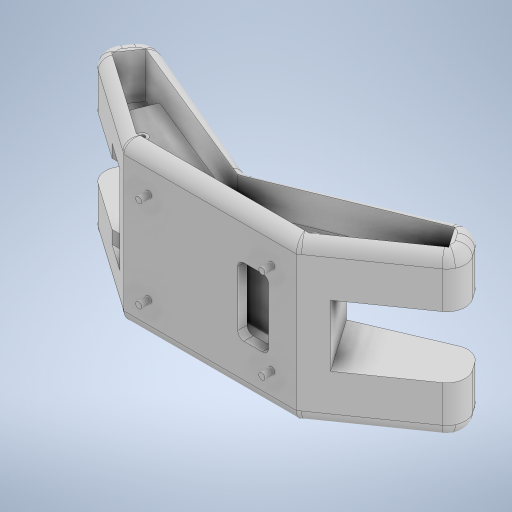
# Autodesk Inventor part: podvozek
Saved by Autodesk Inventor 2024 (Build 280153000, 153)
## iProperties
Created: 2024-03-05
Part Number: podvozek
Material: Všeobecné
Document SubType Name: Modeling
Designer: Game
Density: 1 g/cm^3
Appearance: Výchozí
Author: Game
Autodesk Inventor part; units mm, degrees
ref_plane "XZ Plane" through (0, 0, 0) normal (0, 1, 0) x (-1, 0, 0)
ref_plane "XY Plane" through (0, 0, 0) normal (0, 0, 1) x (1, 0, 0)
sketch "Náčrt1" plane through (0, 0, 0) normal (0, 0, 1) x (1, 0, 0)
  line L0 (-70, 45) -> (70, 45)
  line L1 (70, 45) -> (70, -45)
  line L2 (70, -45) -> (-70, -45)
  line L3 (-70, -45) -> (-70, 45)
  line L4 (-70, 45) -> (70, -45) construction
  line L5 (70, 45) -> (-70, -45) construction
  point P0 (0, 0)
  dimension "d0" = 140
  dimension "d1" = 90
  constraints: 12 end point, 2 midpoint, 2 parallel, 1 horizontal, 1 perpendicular
  measures "d0" distance of L1.end L2.end
  measures "d1" distance of L0.end L1.end
extrude "Vysunutí1" add sketch "Náčrt1" along normal blind 30
sketch "Náčrt2" plane through (-70, -45, 0) normal (-1, 0, 0) x (0, 0, 1)
  line L0 (7.5, 80.5) -> (22.5, 80.5)
  line L1 (22.5, 80.5) -> (22.5, 9.5)
  line L2 (22.5, 9.5) -> (7.5, 9.5)
  line L3 (7.5, 9.5) -> (7.5, 80.5)
  line L4 (7.5, 80.5) -> (22.5, 9.5) construction
  line L5 (22.5, 80.5) -> (7.5, 9.5) construction
  point P0 (0, 45)
  point P1 (15, 45)
  dimension "d4" = 15
  dimension "d5" = 71
  constraints: 12 end point, 2 midpoint, 2 parallel, 1 horizontal, 1 perpendicular
  measures "d4" distance of L1.end L2.end
  measures "d5" distance of L0.end L1.end
extrude "Vysunutí2" cut sketch "Náčrt2" against normal blind 132
sketch "Náčrt3" plane through (0, 0, 30) normal (0, 0, 1) x (1, 0, 0)
  line L0 (50, 37) -> (-50, 37)
  line L1 (-50, 37) -> (-50, -37)
  line L2 (-50, -37) -> (50, -37)
  line L3 (50, -37) -> (50, 37)
  line L4 (50, 37) -> (-50, -37) construction
  line L5 (-50, 37) -> (50, -37) construction
  circle A0 centre (50, -37) radius 2.5
  circle A1 centre (50, 37) radius 2.5
  circle A2 centre (-50, -37) radius 2.5
  circle A3 centre (-50, 37) radius 2.5
  point P0 (0, 0)
  dimension "d8" = 100
  dimension "d9" = 74
  dimension "d10" = 5
  dimension "d13" = 74
  dimension "d16" = 100
  constraints: 12 end point, 4 centre point, 2 horizontal, 2 midpoint, 2 parallel, 1 coincident, 1 perpendicular, 1 vertical, 6 other
  measures "d8" distance of L2.end L1.end
  measures "d9" distance of L1.end L0.end
  measures "d10" diameter of A0
  measures "d13" distance of A0.centre A1.centre
  measures "d16" distance of A0.centre A2.centre
extrude "Vysunutí3" add sketch "Náčrt3" along normal blind 8 contours A3 L1 L0 | L0 L1 A3 | A1 L3 L0 | L0 L3 A1 | A2 L2 L1 | L1 L2 A2 | A0 L2 L3 | L3 L2 A0
sketch "Náčrt7" plane through (-70, 45, 0) normal (0, 1, 0) x (1, 0, 0)
  line L0 (140, 0) -> (140, -30) projected
  line L1 (140, -30) -> (221.9152, 27.3576)
  line L2 (140, -30) -> (240, -30) construction
  line L3 (221.9152, 27.3576) -> (201.84, 56.028)
  line L4 (201.84, 56.028) -> (70, 0)
  line L5 (0, -30) -> (140, -30) projected
  line L6 (0, -30) -> (-81.9152, 27.3576)
  line L7 (0, -30) -> (100, -30) construction
  line L8 (-81.9152, 27.3576) -> (-61.84, 56.028)
  line L9 (-61.84, 56.028) -> (70, 0)
  dimension "d39" = 100
  dimension "d40" = 35
  dimension "d41" = 35
  dimension "d42" = 100
  dimension "d43" = 145
  dimension "d44" = 35
  constraints: 16 end point, 2 equal length, 2 horizontal, 2 perpendicular
  measures "d39" distance of L0.end L1.end
  measures "d40" angle of L2 L1
  measures "d41" distance of L1.end L3.end
  measures "d42" distance of L5.start L6.end
  measures "d43" angle of L7 L6
  measures "d44" distance of L6.end L8.end
extrude "Vysunutí7" add sketch "Náčrt7" along normal blind 20 and the other way blind 110
sketch "Náčrt8" plane through (-70, -65, 30) normal (-0.5735764, 0, 0.819152) x (0.819152, 0, 0.5735764)
  line L0 (-180, 90) -> (-20, 90)
  line L1 (-20, 90) -> (-20, 40)
  line L2 (-20, 40) -> (-180, 40)
  line L3 (-180, 40) -> (-180, 90)
  line L4 (-100, 0) -> (-100, 130) projected
  line L5 (-180, 90) -> (-20, 40) construction
  line L6 (-20, 90) -> (-180, 40) construction
  point P0 (40.1334, 65)
  point P1 (-100, 65)
  point P2 (-100, 40)
  point P3 (-100, 90)
  dimension "d49" = 160
  dimension "d50" = 50
  constraints: 12 end point, 3 midpoint, 2 parallel, 1 horizontal, 1 perpendicular
  measures "d49" distance of L1.end L2.end
  measures "d50" distance of L0.end L1.end
extrude "Vysunutí8" cut sketch "Náčrt8" against normal blind 100
sketch "Náčrt9" plane through (151.9152, -65, -27.3576) normal (0.5735764, 0, 0.819152) x (0.819152, 0, -0.5735764)
  line L0 (-80, 40) -> (80, 40)
  line L1 (80, 40) -> (80, 90)
  line L2 (80, 90) -> (-80, 90)
  line L3 (-80, 90) -> (-80, 40)
  line L4 (0, 130) -> (0, 0) projected
  line L5 (-80, 40) -> (80, 90) construction
  line L6 (80, 40) -> (-80, 90) construction
  point P0 (-140.1334, 65)
  point P1 (0, 65)
  point P2 (0, 40)
  point P3 (0, 90)
  dimension "d53" = 160
  dimension "d54" = 50
  constraints: 12 end point, 3 midpoint, 2 parallel, 1 horizontal, 1 perpendicular
  measures "d53" distance of L2.end L1.end
  measures "d54" distance of L1.end L0.end
extrude "Vysunutí9" cut sketch "Náčrt9" against normal blind 100
ref_plane "Pracovní rovina1" through (-120, 0, 0) normal (1, 0, 0) x (0, 1, 0)
sketch "Náčrt11" plane through (-120, 0, 0) normal (1, 0, 0) x (0, 1, 0)
  line L0 (35.5, 22.5) -> (-35.5, 22.5)
  line L1 (-35.5, 22.5) -> (-35.5, 7.5)
  line L2 (-35.5, 7.5) -> (35.5, 7.5)
  line L3 (35.5, 7.5) -> (35.5, 22.5)
  line L4 (35.5, 22.5) -> (-35.5, 7.5) construction
  line L5 (-35.5, 22.5) -> (35.5, 7.5) construction
  point P0 (0, 0)
  point P1 (0, 15)
  dimension "d58" = 71
  dimension "d59" = 15
  constraints: 12 end point, 2 midpoint, 2 parallel, 1 horizontal, 1 perpendicular
  measures "d58" distance of L2.end L1.end
  measures "d59" distance of L1.end L0.end
extrude "Vysunutí10" cut sketch "Náčrt11" along normal blind 170
sketch "Náčrt12" plane through (-70, -65, 0) normal (0, -1, 0) x (1, 0, 0)
  line L0 (0, 20) -> (-66.8295, -26.7945)
  line L1 (0, 20) -> (81.5838, 20) construction
  line L2 (-66.8295, -26.7945) -> (-55.358, -43.1776)
  line L3 (-55.358, -43.1776) -> (70.0734, 7.5)
  line L4 (-32.1333, 7.5) -> (120, 7.5) projected
  line L5 (-55.358, -43.1776) -> (79.9241, -43.1776) construction
  line L6 (70.0734, 7.5) -> (195.5047, -43.1775)
  line L7 (70.0734, 7.5) -> (205.3554, 7.5) construction
  line L8 (0, 20) -> (140, 20)
  line L9 (140, 20) -> (206.9279, -26.8634)
  line L10 (206.9279, -26.8634) -> (195.5047, -43.1775)
  point P0 (70, 0)
  dimension "d62" = 145
  dimension "d63" = 20
  dimension "d64" = 22
  dimension "d65" = 135.282
  dimension "d66" = 22
  dimension "d67" = 145
  constraints: 20 end point, 4 horizontal, 3 equal length, 2 perpendicular, 1 point on line
  measures "d62" angle of L0 L1
  measures "d63" distance of L0.end L2.end
  measures "d64" angle of L5 L3
  measures "d65" distance of L3.end L6.end
  measures "d66" angle of L6 L7
  measures "d67" angle of L8 L9
extrude "Vysunutí11" cut sketch "Náčrt12" against normal blind 25
sketch "Náčrt13" plane through (-70, 65, 0) normal (0, 1, 0) x (1, 0, 0)
  line L0 (-66.8295, 26.7945) -> (0, -20) projected
  line L1 (0, -20) -> (-66.8295, 26.7945)
  line L2 (70.0734, -7.5) -> (-55.358, 43.1776) projected
  line L3 (-66.8295, 26.7945) -> (-55.358, 43.1776)
  line L4 (-55.358, 43.1776) -> (70, -7.6373)
  line L5 (70, -7.6373) -> (195.5048, 43.1776)
  line L6 (195.5047, 43.1775) -> (70.0734, -7.5) projected
  line L7 (206.9279, 26.8634) -> (195.5047, 43.1775) projected
  line L8 (0, -20) -> (140, -20) projected
  line L9 (206.9279, 26.8634) -> (140, -20)
  line L10 (140, -20) -> (0, -20)
  point P0 (70, 0)
  constraints: 12 end point, 2 collinear, 1 perpendicular, 1 point on line
extrude "Vysunutí12" cut sketch "Náčrt13" against normal blind 25 contours L3 L4 L5 L7 L9 L8 L0
sketch "Náčrt14" plane through (0, 0, 30) normal (0, 0, 1) x (1, 0, 0)
  line L0 (47.5, 27.5) -> (22.5, 27.5)
  line L1 (22.5, 27.5) -> (22.5, -27.5)
  line L2 (22.5, -27.5) -> (47.5, -27.5)
  line L3 (47.5, -27.5) -> (47.5, 27.5)
  line L4 (47.5, 27.5) -> (22.5, -27.5) construction
  line L5 (22.5, 27.5) -> (47.5, -27.5) construction
  point P0 (0, 0)
  point P1 (35, 0)
  dimension "d72" = 25
  dimension "d73" = 55
  constraints: 12 end point, 2 midpoint, 2 parallel, 1 horizontal, 1 perpendicular
  measures "d72" distance of L2.end L1.end
  measures "d73" distance of L1.end L0.end
extrude "Vysunutí13" cut sketch "Náčrt14" against normal blind 20
fillet "Zaoblení1" radius 5 4 edges at (47.5, 27.5, 26.25) (47.5, -27.5, 26.25) (22.5, 27.5, 26.25) (22.5, -27.5, 26.25)
fillet "Zaoblení2" radius 10 1 edges at (0, 0, 0)
sketch "Náčrt17" plane through (-70, -40, 0) normal (0, -1, 0) x (1, 0, 0)
  line L0 (-55.358, -43.1776) -> (-66.8295, -26.7945) projected
  line L1 (70.0734, 7.5) -> (-55.358, -43.1776) projected
  line L2 (-66.8295, -26.7945) -> (-55.358, -43.1776)
  line L3 (-55.358, -43.1776) -> (-36.8143, -35.6854)
  line L4 (-36.8143, -35.6854) -> (-46.2332, -12.3728)
  line L5 (-66.8295, -26.7945) -> (0, 20) projected
  line L6 (-46.2332, -12.3728) -> (-66.8295, -26.7945)
  line L7 (195.5047, -43.1775) -> (70.0734, 7.5) projected
  line L8 (195.5047, -43.1775) -> (176.961, -35.6854)
  line L9 (206.9279, -26.8634) -> (195.5047, -43.1775) projected
  line L10 (195.5047, -43.1775) -> (206.9279, -26.8634)
  line L11 (206.9279, -26.8634) -> (140, 20) projected
  line L12 (176.961, -35.6854) -> (187.1443, -10.4809)
  line L13 (176.961, -35.6854) -> (204.1449, -35.6854) construction
  line L14 (206.9279, -26.8634) -> (186.3476, -12.4529)
  point P0 (70, 0)
  dimension "d78" = 20
  dimension "d79" = 90
  dimension "d82" = 20
  dimension "d83" = 68
  constraints: 18 end point, 5 point on line, 1 collinear, 1 equal length, 1 horizontal, 1 perpendicular
  measures "d78" distance of L0.start L3.end
  measures "d79" angle of L4 L3
  measures "d82" distance of L7.start L8.end
  measures "d83" angle of L13 L12
extrude "Vysunutí14" cut sketch "Náčrt17" against normal blind 12
sketch "Náčrt18" plane through (-70, 40, 0) normal (0, 1, 0) x (1, 0, 0)
  line L0 (70, -7.6373) -> (195.5047, 43.1775) projected
  line L1 (195.5047, 43.1775) -> (176.9665, 35.6717)
  line L2 (176.9665, 35.6717) -> (186.3631, 12.4638)
  line L3 (206.9279, 26.8634) -> (140, -20) projected
  line L4 (186.3631, 12.4638) -> (206.9279, 26.8634)
  line L5 (206.9279, 26.8634) -> (195.5047, 43.1775)
  line L6 (-55.358, 43.1776) -> (70, -7.6373) projected
  line L7 (-55.358, 43.1776) -> (-36.8229, 35.6642)
  line L8 (-55.358, 43.1776) -> (70, -7.6373) projected
  line L9 (-36.8229, 35.6642) -> (-46.2574, 12.3898)
  line L10 (0, -20) -> (-66.8295, 26.7945) projected
  line L11 (-46.2574, 12.3898) -> (-66.8295, 26.7945)
  line L12 (-66.8295, 26.7945) -> (-55.358, 43.1776)
  point P0 (70, 0)
  dimension "d84" = 20
  dimension "d85" = 90
  dimension "d86" = 20
  dimension "d87" = 90
  constraints: 16 end point, 4 point on line, 2 collinear, 2 perpendicular
  measures "d84" distance of L0.end L1.end
  measures "d85" angle of L2 L1
  measures "d86" distance of L6.start L7.end
  measures "d87" angle of L7 L9
extrude "Vysunutí15" cut sketch "Náčrt18" against normal blind 12
sketch "Náčrt19" plane through (-70, -40, 0) normal (0, -1, 0) x (1, 0, 0)
  circle A0 centre (105, 15) radius 4
  point P0 (70, 0)
  dimension "d90" = 8
  constraints: 1 centre point
  measures "d90" diameter of A0
extrude "Vysunutí16" cut sketch "Náčrt19" against normal blind 100
fillet "Zaoblení3" radius 15 8 edges at (-151.9152, -45, -27.3576) (-131.84, -45, -56.028) (-151.9152, 45, -27.3576) (-131.84, 45, -56.028) (131.84, 45, -56.028) (131.84, -45, -56.028) (151.9152, -45, -27.3576) (151.9152, 45, -27.3576)
fillet "Zaoblení4" radius 10 24 edges at (0, 65, 30) (-145.7964, 65, -28.4366) (-141.0608, 65, -42.8593) (-130.6544, 65, -51.8898) (-62.2836, 65, -26.4686) (0, 65, -0.8655) (62.2836, 65, -26.4686) (130.6544, 65, -51.8898) (141.0608, 65, -42.8593) (145.7964, 65, -28.4366) (104.814, 65, 5.623) (-104.814, 65, 5.623) (-145.7964, -65, -28.4366) (-141.0608, -65, -42.8593) (-130.6544, -65, -51.8898) (-62.2836, -65, -26.4686) (0, -65, -0.8655) (62.2836, -65, -26.4686) (130.6544, -65, -51.8898) (141.0608, -65, -42.8593) (145.7964, -65, -28.4366) (104.814, -65, 5.623) (-104.814, -65, 5.623) (0, -65, 30)
sketch "Náčrt20" plane through (-70, -40, 0) normal (0, -1, 0) x (1, 0, 0)
  circle A0 centre (0, 15) radius 4
  circle A1 centre (140, 15) radius 4
  line L0 (4, 15) -> (4, 20)
  line L1 (0, 20) -> (140, 20) projected
  line L2 (-4, 15) -> (-5.0333, 16.4757)
  line L3 (-46.2332, -12.3728) -> (0, 20) projected
  line L4 (136, 15) -> (136, 20)
  line L5 (-10.7111, 22.5) -> (120, 22.5) projected
  line L6 (136, 20) -> (140, 20)
  line L7 (144, 15) -> (145.0333, 16.4757)
  line L8 (140, 20) -> (186.3476, -12.4529) projected
  line L9 (-5.0333, 16.4757) -> (0, 20)
  circle A2 centre (0, 15) radius 2
  circle A3 centre (140, 15) radius 2
  point P0 (70, 0)
  dimension "d95" = 8
  dimension "d96" = 8
  dimension "d97" = 4
  dimension "d98" = 4
  constraints: 12 end point, 4 centre point, 4 point on circle, 3 point on line, 2 coincident, 2 perpendicular, 1 collinear, 1 tangent, 1 vertical
  measures "d95" diameter of A0
  measures "d96" diameter of A1
  measures "d97" diameter of A2
  measures "d98" diameter of A3
extrude "Vysunutí17" add sketch "Náčrt20" along normal blind 20
sketch "Náčrt21" plane through (-70, 40, 0) normal (0, 1, 0) x (1, 0, 0)
  circle A0 centre (140, -15) radius 2 projected
  circle A1 centre (140, -15) radius 4
  circle A2 centre (0, -15) radius 2 projected
  circle A3 centre (0, -15) radius 4
  line L0 (4, -20) -> (136, -20) projected
  line L1 (4, -15) -> (4, -20)
  line L2 (4, -20) -> (0, -20)
  line L3 (136, -20) -> (136, -15) projected
  line L4 (136, -15) -> (136, -20)
  line L5 (136, -20) -> (140, -20) projected
  line L6 (136, -20) -> (140, -20)
  line L7 (144, -15) -> (145.0333, -16.4757) projected
  line L8 (144, -15) -> (145.0333, -16.4757)
  line L9 (145.0333, -16.4757) -> (140, -20)
  line L10 (-5.0333, -16.4757) -> (-4, -15) projected
  line L11 (-4, -15) -> (-5.0333, -16.4757)
  line L12 (-5.0333, -16.4757) -> (0, -20)
  circle A4 centre (140, -15) radius 2
  circle A5 centre (0, -15) radius 2
  point P0 (70, 0)
  constraints: 16 end point, 4 centre point, 4 coincident, 4 collinear, 3 perpendicular, 2 concentric, 2 point on circle, 1 tangent, 1 vertical
extrude "Vysunutí18" add sketch "Náčrt21" along normal blind 20
